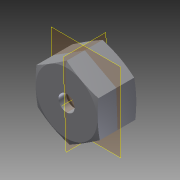
# Autodesk Inventor part: Pneumatics_VIAIR_Fitting_01
Saved by Autodesk Inventor 2014 (Build 180170000, 170)
## iProperties
Created: 2011-11-29
Part Number: Pneumatics_VIAIR_Fitting_01
Material: Generic
Document SubType Name: Modeling
Designer: Phillip
Density: 1 g/cm^3
Appearance: Default
Author: Phillip
Autodesk Inventor part; units mm, degrees
ref_plane "YZ Plane" through (0, 0, 0) normal (1, 0, 0) x (0, 1, 0)
ref_plane "XZ Plane" through (0, 0, 0) normal (0, 1, 0) x (-1, 0, 0)
ref_plane "Work Plane3" through (-1.6844, 0, -2.032) normal (0, 0, 1) x (0.9993818, 0.0351571, 0)
sketch "Sketch6" plane through (-1.6844, 0, -2.032) normal (0, 0, 1) x (0.9993818, 0.0351571, 0)
  circle A0 centre (0, 0) radius 6.35
  line L0 (0, 7.3323) -> (6.35, 3.6662)
  line L1 (6.35, 3.6662) -> (6.35, -3.6662)
  line L2 (6.35, -3.6662) -> (0, -7.3323)
  line L3 (0, -7.3323) -> (-6.35, -3.6662)
  line L4 (-6.35, -3.6662) -> (-6.35, 3.6662)
  line L5 (-6.35, 3.6662) -> (0, 7.3323)
  point P0 (1.6833, -0.0592)
  point P1 (0, 7.8524)
  dimension "d5" = 12.7
  constraints: 12 end point, 2 coincident, 1 centre point, 1 tangent, 1 vertical alignment, 15 other
  measures "d5" diameter of A0
extrude "Extrusion2" add sketch "Sketch6" along normal blind 7.9375
sketch "Sketch7" plane through (-1.6844, 0, -2.032) normal (0, 0, -1) x (-0.9993818, -0.0351571, 0)
  circle A0 centre (-0.0028, 0.0799) radius 4.3656 projected
  point P0 (-1.6833, -0.0592)
extrude "Extrusion3" cut sketch "Sketch7" against normal blind 6.35 draft -1.783
sketch "Sketch8" plane through (-1.6844, 0, 5.9055) normal (0, 0, 1) x (0.9993818, 0.0351571, 0)
  circle A0 centre (0.0028, 0.0799) radius 1.651 projected
  point P0 (1.6833, -0.0592)
extrude "Extrusion4" cut sketch "Sketch8" against normal through all
thread "Thread1" size "1/8" designation "1/8 - 27 NPT" standard "NPT for PVC Pipe and Fitting" length 9.9568
ref_plane "Work Plane4" through (-1.9422, 7.3278, -2.032) normal (0.9993818, 0.0351571, 0) x (0, 0, 1)
sketch "Sketch9" plane through (-1.9422, 7.3278, -2.032) normal (0.9993818, 0.0351571, 0) x (0, 0, 1)
  line L0 (7.9375, 13.5217) -> (7.593, 14.6647)
  line L1 (7.593, 14.6647) -> (7.9375, 13.5217)
  line L2 (7.593, 14.6647) -> (7.9375, 14.6647)
  line L3 (7.9375, 14.6647) -> (7.9375, 13.5217)
  line L4 (9.525, 7.2525) -> (-1.5875, 7.2525) projected
  point P0 (2.032, 7.3916)
  dimension "d13" = 1.143
  constraints: 8 end point, 1 collinear, 1 horizontal, 1 vertical
  measures "d13" distance of L2.end L0.start
revolve "Revolution2" cut sketch "Sketch9" angle 360 about axis through (-1.6872, 0.0798, 5.9055) along (0, 0, -1)
ref_plane "Work Plane5" through (-1.6872, 0.0798, 1.9367) normal (0, 0, 1) x (1, 0, 0)
mirror "Mirror1" about plane through (-1.6872, 0.0798, 1.9367) normal (0, 0, 1) of "Revolution2"
body "Solid2"
